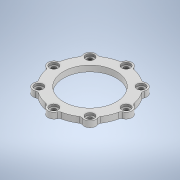
# Autodesk Inventor part: Outer_flange
Saved by Autodesk Inventor 2020.4 (Build 244396000, 396)
## iProperties
Created: 2021-09-25
Part Number: Outer_flange
Material: アルミニウム 2014-T4
Document SubType Name: Modeling
Designer: Masato Kubotera
Density: 2.8 g/cm^3
Appearance: 滑らか - 淡い灰色
Mass: 11.7454 g
Surface Area: 38.0772 cm^2
Volume: 4.19478 cm^3
Author: Masato Kubotera
Keywords: A2017 T4
Autodesk Inventor part; units mm, degrees
ref_plane "YZ Plane" through (0, 0, 0) normal (1, 0, 0) x (0, 1, 0)
ref_plane "XZ Plane" through (0, 0, 0) normal (0, 1, 0) x (-1, 0, 0)
ref_plane "XY Plane" through (0, 0, 0) normal (0, 0, 1) x (1, 0, 0)
derived "Outer_support_stand.ipt"
sketch "スケッチ1" plane through (0, 0, 0) normal (0, 0, 1) x (1, 0, 0)
  line L0 (-62, 30.75) -> (62, 30.75)
  line L1 (62, -30.75) -> (-62, -30.75)
  line L2 (-62, 30.75) -> (62, -30.75) construction
  line L3 (62, 30.75) -> (-62, -30.75) construction
  line L4 (0, 30.75) -> (0, -30.75) construction
  circle A0 centre (-44, 2.25) radius 10.5 construction
  line L5 (-57.5, 1.25) -> (-30.5, 1.25) construction
  line L6 (-30.5, 1.25) -> (-30.5, -25.75) construction
  line L7 (-30.5, -25.75) -> (-57.5, -25.75) construction
  line L8 (-57.5, -25.75) -> (-57.5, 1.25) construction
  line L9 (-44, 1.25) -> (-44, -25.75) construction
  line L10 (-57.5, -12.25) -> (-30.5, -12.25) construction
  circle A1 centre (-57.5, 1.25) radius 1.35
  circle A2 centre (-57.5, -25.75) radius 1.35
  circle A3 centre (-30.5, 1.25) radius 1.35
  circle A4 centre (-30.5, -25.75) radius 1.35
  line L11 (-27.5, 21.75) -> (-22.5, 21.75) construction
  line L12 (-22.5, 21.75) -> (-22.5, 11.75) construction
  line L13 (-22.5, 11.75) -> (-27.5, 11.75) construction
  line L14 (-27.5, 11.75) -> (-27.5, 21.75) construction
  line L15 (-27.5, 21.75) -> (-22.5, 11.75) construction
  line L16 (-22.5, 21.75) -> (-27.5, 11.75) construction
  line L17 (-27.51, 21.76) -> (-22.49, 21.76)
  line L18 (-22.49, 21.76) -> (-22.49, 11.74)
  line L19 (-22.49, 11.74) -> (-27.51, 11.74)
  line L20 (-27.51, 11.74) -> (-27.51, 21.76)
  line L21 (-27.51, 21.76) -> (-22.49, 11.74) construction
  line L22 (-22.49, 21.76) -> (-27.51, 11.74) construction
  line L23 (-27.51, 16.75) -> (-22.49, 16.75) construction
  line L24 (-25, 21.76) -> (-25, 11.74) construction
  arc A5 (-27.51, 21.76) -> (-27.51, 19.66) centre (-27.51, 20.71) ccw
  arc A6 (-22.49, 19.66) -> (-22.49, 21.76) centre (-22.49, 20.71) ccw
  arc A7 (-27.51, 13.84) -> (-27.51, 11.74) centre (-27.51, 12.79) ccw
  arc A8 (-22.49, 11.74) -> (-22.49, 13.84) centre (-22.49, 12.79) ccw
  circle A9 centre (-25, 27.75) radius 1.55
  line L25 (-27.5, -9.25) -> (-22.5, -9.25) construction
  line L26 (-22.5, -9.25) -> (-22.5, -21.75) construction
  line L27 (-22.5, -21.75) -> (-27.5, -21.75) construction
  line L28 (-27.5, -21.75) -> (-27.5, -9.25) construction
  line L29 (-27.5, -9.25) -> (-22.5, -21.75) construction
  line L30 (-22.5, -9.25) -> (-27.5, -21.75) construction
  line L31 (-27.51, -9.24) -> (-22.49, -9.24)
  line L32 (-22.49, -9.24) -> (-22.49, -21.76)
  line L33 (-22.49, -21.76) -> (-27.51, -21.76)
  line L34 (-27.51, -21.76) -> (-27.51, -9.24)
  line L35 (-27.51, -9.24) -> (-22.49, -21.76) construction
  line L36 (-22.49, -9.24) -> (-27.51, -21.76) construction
  line L37 (-27.51, -15.5) -> (-22.49, -15.5) construction
  line L38 (-25, -9.24) -> (-25, -21.76) construction
  arc A10 (-27.51, -9.24) -> (-27.51, -11.34) centre (-27.51, -10.29) ccw
  arc A11 (-22.49, -11.34) -> (-22.49, -9.24) centre (-22.49, -10.29) ccw
  arc A12 (-22.49, -21.76) -> (-22.49, -19.66) centre (-22.49, -20.71) ccw
  arc A13 (-27.51, -19.66) -> (-27.51, -21.76) centre (-27.51, -20.71) ccw
  circle A14 centre (-25, -27.75) radius 1.55
  circle A15 centre (-44, 2.25) radius 11
  line L39 (62, 2.25) -> (-62, 2.25) construction
  line L40 (-60, 14.25) -> (-28, 14.25) construction
  line L41 (-28, 14.25) -> (-28, -28.75) construction
  line L42 (-28, -28.75) -> (-60, -28.75) construction
  line L43 (-60, -28.75) -> (-60, 14.25) construction
  line L44 (-60, 14.25) -> (-28, -28.75) construction
  line L45 (-28, 14.25) -> (-60, -28.75) construction
  line L46 (-62, 30.75) -> (-62, -30.75) construction
  line L47 (62, 30.75) -> (62, -30.75) construction
  circle A16 centre (-44, 2.25) radius 12.5 construction
  circle A17 centre (-44, 2.25) radius 20.5 construction
  circle A18 centre (-44, 2.25) radius 28.5 construction
  circle A19 centre (-44, 26.75) radius 2.2 construction
  circle A20 centre (-61.3241, 19.5741) radius 2.2 construction
  circle A21 centre (-68.5, 2.25) radius 2.2 construction
  circle A22 centre (-61.3241, -15.0741) radius 2.2 construction
  circle A23 centre (-44, -22.25) radius 2.2 construction
  circle A24 centre (-26.6759, -15.0741) radius 2.2 construction
  circle A25 centre (-19.5, 2.25) radius 2.2 construction
  circle A26 centre (-26.6759, 19.5741) radius 2.2 construction
  line L48 (-62, -21.122) -> (-62, -30.75)
  circle A27 centre (57.5, 1.25) radius 1.35
  circle A28 centre (57.5, -25.75) radius 1.35
  circle A29 centre (30.5, 1.25) radius 1.35
  circle A30 centre (30.5, -25.75) radius 1.35
  line L49 (27.51, 21.76) -> (22.49, 21.76)
  line L50 (22.49, 21.76) -> (22.49, 11.74)
  line L51 (22.49, 11.74) -> (27.51, 11.74)
  line L52 (27.51, 11.74) -> (27.51, 21.76)
  arc A31 (27.51, 19.66) -> (27.51, 21.76) centre (27.51, 20.71) ccw
  arc A32 (22.49, 21.76) -> (22.49, 19.66) centre (22.49, 20.71) ccw
  arc A33 (22.49, 13.84) -> (22.49, 11.74) centre (22.49, 12.79) ccw
  arc A34 (27.51, 11.74) -> (27.51, 13.84) centre (27.51, 12.79) ccw
  circle A35 centre (25, 27.75) radius 1.55
  arc A36 (27.51, -21.76) -> (27.51, -19.66) centre (27.51, -20.71) ccw
  line L53 (22.49, -21.76) -> (27.51, -21.76)
  arc A37 (22.49, -19.66) -> (22.49, -21.76) centre (22.49, -20.71) ccw
  line L54 (27.51, -21.76) -> (27.51, -9.24)
  line L55 (22.49, -9.24) -> (22.49, -21.76)
  circle A38 centre (25, -27.75) radius 1.55
  arc A39 (22.49, -9.24) -> (22.49, -11.34) centre (22.49, -10.29) ccw
  line L56 (27.51, -9.24) -> (22.49, -9.24)
  arc A40 (27.51, -11.34) -> (27.51, -9.24) centre (27.51, -10.29) ccw
  circle A41 centre (44, 2.25) radius 11
  circle A42 centre (44, 26.75) radius 2.2
  circle A43 centre (61.3241, 19.5741) radius 2.2
  circle A44 centre (68.5, 2.25) radius 2.2
  circle A45 centre (61.3241, -15.0741) radius 2.2
  circle A46 centre (44, -22.25) radius 2.2
  circle A47 centre (26.6759, -15.0741) radius 2.2
  circle A48 centre (19.5, 2.25) radius 2.2
  circle A49 centre (26.6759, 19.5741) radius 2.2
  line L57 (62, -21.122) -> (62, -30.75)
  circle A50 centre (-44, 2.25) radius 20.51
  circle A51 centre (-44, 2.25) radius 18.5
  circle A52 centre (-44, 2.25) radius 28.5
  circle A53 centre (-44, 26.75) radius 1.55
  circle A54 centre (-61.3241, 19.5741) radius 1.55
  circle A55 centre (-68.5, 2.25) radius 1.55
  circle A56 centre (-61.3241, -15.0741) radius 1.55
  circle A57 centre (-44, -22.25) radius 1.55
  circle A58 centre (-26.6759, -15.0741) radius 1.55
  circle A59 centre (-19.5, 2.25) radius 1.55
  circle A60 centre (-26.6759, 19.5741) radius 1.55
  line L58 (-68.5, 2.25) -> (-73.5, 2.25) construction
  circle A61 centre (-26.6759, -15.0741) radius 7.2 construction
  circle A62 centre (-44, 2.25) radius 24.5 construction
  circle A63 centre (-44, 26.75) radius 3.05
  circle A64 centre (-61.3241, 19.5741) radius 3.05
  circle A65 centre (-68.5, 2.25) radius 3.05
  circle A66 centre (-44, -22.25) radius 3.05
  circle A67 centre (-26.6759, -15.0741) radius 3.05
  circle A68 centre (-19.5, 2.25) radius 3.05
  circle A69 centre (-26.6759, 19.5741) radius 3.05
  circle A70 centre (-61.3241, -15.0741) radius 3.05
  circle A71 centre (-44, 2.25) radius 17.9
  circle A72 centre (-44, 26.75) radius 2.9
  circle A73 centre (-61.3241, 19.5741) radius 2.9
  circle A74 centre (-68.5, 2.25) radius 2.9
  circle A75 centre (-61.3241, -15.0741) radius 2.9
  circle A76 centre (-44, -22.25) radius 2.9
  circle A77 centre (-26.6759, -15.0741) radius 2.9
  circle A78 centre (-19.5, 2.25) radius 2.9
  circle A79 centre (-26.6759, 19.5741) radius 2.9
  circle A80 centre (-30.5, -25.75) radius 2.4
  arc A81 (-44, 30.75) -> (-47.969, 27.2469) centre (-44, 26.75) ccw
  arc A82 (-58.8689, 22.732) -> (-64.1525, 22.4025) centre (-61.3241, 19.5741) ccw
  arc A83 (-47.969, 27.2469) -> (-58.8689, 22.732) centre (-44, 2.25) ccw
  arc A84 (-64.1525, 22.4025) -> (-64.482, 17.1189) centre (-61.3241, 19.5741) ccw
  arc A85 (-64.482, 17.1189) -> (-68.9969, 6.219) centre (-44, 2.25) ccw
  arc A86 (-68.9969, 6.219) -> (-72.5, 2.25) centre (-68.5, 2.25) ccw
  arc A87 (-72.5, 2.25) -> (-68.9969, -1.719) centre (-68.5, 2.25) ccw
  arc A88 (-68.9969, -1.719) -> (-64.482, -12.6189) centre (-44, 2.25) ccw
  arc A89 (-64.482, -12.6189) -> (-64.1525, -17.9025) centre (-61.3241, -15.0741) ccw
  arc A90 (-64.1525, -17.9025) -> (-58.8689, -18.232) centre (-61.3241, -15.0741) ccw
  arc A91 (-58.8689, -18.232) -> (-47.969, -22.7469) centre (-44, 2.25) ccw
  arc A92 (-47.969, -22.7469) -> (-44, -26.25) centre (-44, -22.25) ccw
  arc A93 (-44, -26.25) -> (-40.031, -22.7469) centre (-44, -22.25) ccw
  arc A94 (-40.031, -22.7469) -> (-29.1311, -18.232) centre (-44, 2.25) ccw
  arc A95 (-29.1311, -18.232) -> (-23.8475, -17.9025) centre (-26.6759, -15.0741) ccw
  arc A96 (-23.8475, -17.9025) -> (-23.518, -12.6189) centre (-26.6759, -15.0741) ccw
  arc A97 (-23.518, -12.6189) -> (-19.0031, -1.719) centre (-44, 2.25) ccw
  arc A98 (-19.0031, -1.719) -> (-15.5, 2.25) centre (-19.5, 2.25) ccw
  arc A99 (-15.5, 2.25) -> (-19.0031, 6.219) centre (-19.5, 2.25) ccw
  arc A100 (-19.0031, 6.219) -> (-23.518, 17.1189) centre (-44, 2.25) ccw
  arc A101 (-23.518, 17.1189) -> (-23.8475, 22.4025) centre (-26.6759, 19.5741) ccw
  arc A102 (-23.8475, 22.4025) -> (-29.1311, 22.732) centre (-26.6759, 19.5741) ccw
  arc A103 (-29.1311, 22.732) -> (-40.031, 27.2469) centre (-44, 2.25) ccw
  arc A104 (-40.031, 27.2469) -> (-44, 30.75) centre (-44, 26.75) ccw
  arc A105 (-48.9902, 27.0632) -> (-58.017, 23.3242) centre (-44, 2.25) ccw
  arc A106 (-41, 30.75) -> (-48.9902, 27.0632) centre (-44, 26.75) ccw
  arc A107 (-58.017, 23.3242) -> (-65.0742, 16.267) centre (-61.3241, 19.5741) ccw
  arc A108 (-65.0742, 16.267) -> (-68.8132, 7.2402) centre (-44, 2.25) ccw
  arc A109 (-68.8132, 7.2402) -> (-68.8132, -2.7402) centre (-68.5, 2.25) ccw
  arc A110 (-68.8132, -2.7402) -> (-65.0742, -11.767) centre (-44, 2.25) ccw
  arc A111 (-65.0742, -11.767) -> (-62, -20.0282) centre (-61.3241, -15.0741) ccw
  line L59 (-62, -20.0282) -> (-62, -21.122)
  arc A112 (58.017, 23.3242) -> (48.9902, 27.0632) centre (44, 2.25) ccw
  arc A113 (48.9902, 27.0632) -> (41, 30.75) centre (44, 26.75) ccw
  arc A114 (65.0742, 16.267) -> (58.017, 23.3242) centre (61.3241, 19.5741) ccw
  arc A115 (68.8132, 7.2402) -> (65.0742, 16.267) centre (44, 2.25) ccw
  arc A116 (68.8132, -2.7402) -> (68.8132, 7.2402) centre (68.5, 2.25) ccw
  arc A117 (65.0742, -11.767) -> (68.8132, -2.7402) centre (44, 2.25) ccw
  arc A118 (62, -20.0282) -> (65.0742, -11.767) centre (61.3241, -15.0741) ccw
  line L60 (62, -20.0282) -> (62, -21.122)
  line L61 (19.5, 27.75) -> (-19.5, 27.75)
  line L62 (-19.5, 27.75) -> (-19.5, 7.25)
  circle A119 centre (-25, 27.75) radius 2.75 construction
  line L63 (-14.7303, 3.75) -> (14.7303, 3.75)
  arc A120 (-14.7303, 3.75) -> (-19.5, 7.25) centre (-19.5, 2.25) ccw
  line L64 (19.5, 27.75) -> (19.5, 7.25)
  arc A121 (19.5, 7.25) -> (14.7303, 3.75) centre (19.5, 2.25) ccw
  line L65 (-14.7303, 0.75) -> (14.7303, 0.75)
  arc A122 (-19.5, -2.75) -> (-14.7303, 0.75) centre (-19.5, 2.25) ccw
  arc A123 (14.7303, 0.75) -> (19.5, -2.75) centre (19.5, 2.25) ccw
  line L66 (-19.5, -2.75) -> (-19.5, -27.75)
  line L67 (-19.5, -27.75) -> (19.5, -27.75)
  line L68 (19.5, -27.75) -> (19.5, -2.75)
  point P0 (0, 0)
  point P1 (-25, 16.75)
  point P2 (-25, -15.5)
  point P3 (-44, -7.25)
  point P4 (-23.8475, 22.4025)
  point P5 (-44, 30.75)
  point P6 (-64.1525, -17.9025)
  point P7 (-44, -26.25)
  point P8 (-23.8475, -17.9025)
  point P9 (-15.5, 2.25)
  dimension "d1" = 35.8
  dimension "d7" = 5.8
  dimension "d8" = 5.8
  dimension "d9" = 5.8
  dimension "d10" = 5.8
  dimension "d11" = 5.8
  dimension "d12" = 5.8
  dimension "d13" = 5.8
  dimension "d14" = 5.8
  measures "d1" diameter of A71
  measures "d7" diameter of A72
  measures "d8" diameter of A73
  measures "d9" diameter of A74
  measures "d10" diameter of A75
  measures "d11" diameter of A76
  measures "d12" diameter of A77
  measures "d13" diameter of A78
  measures "d14" diameter of A79
extrude "押し出し1" add sketch "スケッチ1" along normal blind 4 contours A104 A103 A102 A101 L17 A69 L20 A50 A10 L34 A67 A95 A94 A93 A92 A91 A90 A89 A88 A87 A86 A85 A84 A82 A83 A81 | A101 A100 L18 L19 A50 L20 A69 L17 | A69 L20 A79 L17 | L17 A79 L20 A69 | A100 L62 A120 A99 A98 A97 A122 L66 A11 L31 A50 L19 A8 L18 | A50 L19 L20 | L20 A7 L19 A50 L31 A10 | A8 L18 | A100 A120 L62 | L20 A7 | A50 L34 A10 | A10 L34 A50 | L31 A50 L34 | L34 A50 L31 L32 A97 A96 A95 A67 | A67 L34 A77 | L34 A77 A67 | A97 L66 A122 | A11 A97 L32 | A51 | A63 | A64 | A65 | A66 | A68 | A70 picked at (-22.3943, -10.3142)
extrude "押し出し2" add sketch "スケッチ1" along normal blind 2.5 contours A79 L20 A60 L17 | L17 A5 A60 L20 A79 | L20 A60 A5 | A77 L34 A58 | L34 A58 A77 | A72 | A73 | A74 | A75 | A76 | A78 picked at (-27.8233, 21.0216)
fillet "フィレット1" radius 2 16 edges at (-58.8689, 22.732, 2) (-40.031, 27.2469, 2) (-47.969, 27.2469, 2) (-29.1311, 22.732, 2) (-23.518, 17.1189, 2) (-19.0031, -1.719, 2) (-23.518, -12.6189, 2) (-40.031, -22.7469, 2) (-19.0031, 6.219, 2) (-64.482, 17.1189, 2) (-68.9969, 6.219, 2) (-68.9969, -1.719, 2) (-64.482, -12.6189, 2) (-58.8689, -18.232, 2) (-47.969, -22.7469, 2) (-29.1311, -18.232, 2)
equation "\"d8\" = d7"
equation "\"d9\" = d7"
equation "\"d10\" = d7"
equation "\"d11\" = d7"
equation "\"d12\" = d7"
equation "\"d13\" = d7"
equation "\"d14\" = d7"
